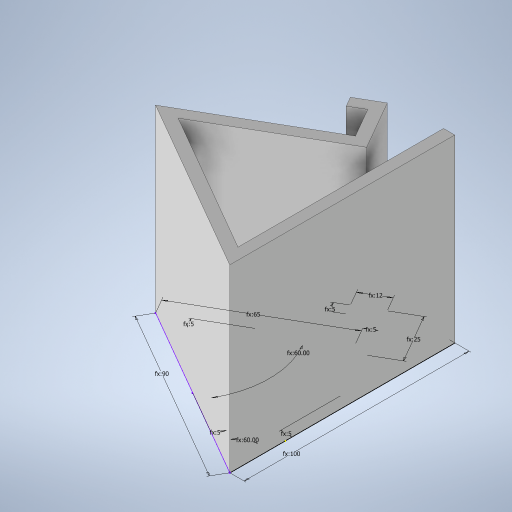
# Autodesk Inventor part: phonestand2DSketch_afterExtrusion
Saved by Autodesk Inventor 2024.2 (Build 282272000, 272)
## iProperties
Created: 2025-02-05
Part Number: phonestand2DSketch_afterExtrusion
Material: Generic
Document SubType Name: Modeling
Designer: veillettem
Density: 1 g/cm^3
Appearance: Default
Author: veillettem
Autodesk Inventor part; units mm, degrees
ref_plane "YZ Plane" through (0, 0, 0) normal (1, 0, 0) x (0, 1, 0)
ref_plane "XZ Plane" through (0, 0, 0) normal (0, 1, 0) x (-1, 0, 0)
ref_plane "XY Plane" through (0, 0, 0) normal (0, 0, 1) x (1, 0, 0)
sketch "PhoneStandProfile" plane through (0, 0, 0) normal (0, 1, 0) x (-1, 0, 0)
  line L0 (5, -75.5038) -> (0, -75.5038)
  line L1 (0, -75.5038) -> (0, 24.4962)
  line L2 (0, 24.4962) -> (77.9423, -20.5038)
  line L3 (77.9423, -20.5038) -> (21.6506, -53.0038)
  line L4 (29.1506, -65.9942) -> (35.2128, -62.4942)
  line L5 (37.7128, -66.8243) -> (27.3205, -72.8243)
  line L6 (27.3205, -72.8243) -> (14.8205, -51.1737)
  line L7 (14.8205, -51.1737) -> (67.9423, -20.5038)
  line L8 (67.9423, -20.5038) -> (5, 15.8359)
  line L9 (5, 15.8359) -> (5, -75.5038)
  line L10 (21.6506, -53.0038) -> (29.1506, -65.9942)
  line L11 (35.2128, -62.4942) -> (37.7128, -66.8243)
  point P0 (0, 0)
  point P1 (0, 24.4962)
  point P2 (77.9423, -20.5038)
  point P3 (5, -29.8339)
  point P4 (38.9711, 1.9962)
  point P5 (49.7965, -36.7538)
  point P6 (21.0705, -61.999)
  point P7 (2.5, -75.5038)
  point P8 (67.9423, -20.5038)
  point P9 (77.9423, -20.5038)
  point P10 (5, 15.8359)
  point P11 (0, 24.4962)
  point P12 (0, 19.6715)
  point P13 (5, 15.8359)
  point P14 (0, 18.7227)
  point P15 (67.9423, -20.5038)
  dimension "angleBackAndSupport" = 60
  dimension "angleBaseAndBack" = 60
  dimension "baseThickness" = 5
  dimension "backThickness" = 5
  dimension "supportThickness" = 5
  dimension "lipThickness" = 5
  dimension "ledgeThickness" = 5
  dimension "ledgeLength" = 25
  dimension "baseL" = 100
  dimension "backL" = 90
  dimension "supportL" = 65
  dimension "lipH" = 12
  constraints: 24 end point, 5 midpoint, 5 point on line, 4 parallel, 4 vertical, 3 perpendicular, 22 other
  measures "angleBackAndSupport" angle of L7 L8
  measures "angleBaseAndBack" angle of L9 L8
  measures "baseThickness" distance from line of L1 point (5, -29.834)
  measures "backThickness" distance from line of L8 point (38.971, 1.996)
  measures "supportThickness" distance from line of point (49.796, -36.754) L7
  measures "lipThickness" distance between parallel lines of L5 L4
  measures "ledgeThickness" distance between parallel lines of L6 L10
  measures "ledgeLength" distance between parallel lines of L5 L7
  measures "baseL" vertical distance of point (0, 24.496) point (2.5, -75.504)
  measures "backL" distance of point (0, 24.496) point (77.942, -20.504)
  measures "supportL" distance of point (77.942, -20.504) L3.end
  measures "lipH" distance of L5.start L5.end
extrude "MainBody" add sketch "PhoneStandProfile" along normal blind 80
sketch "Rectangle" plane through (-37.7128, 0, -66.8243) normal (-0.5, 0, -0.866) x (-0.866, 0, 0.5)
  line L0 (-12, 0) -> (-12, 80) projected
  line L1 (0.2233, 48) -> (-12, 48)
  line L2 (-12, 48) -> (-12, 32)
  line L3 (-12, 32) -> (0.2233, 32)
  line L4 (0.2233, 32) -> (0.2233, 48)
  line L5 (-12, 0) -> (0, 0) projected
  line L6 (-12, 80) -> (0, 80) projected
  point P0 (0.7519, 0)
  point P1 (-6, 80)
  point P2 (-5.8884, 48)
  point P3 (-12, 48)
  dimension "distanceFromRightEdge" = 32
  dimension "distanceFromLeftEdge" = 32
  constraints: 8 end point, 2 midpoint, 2 parallel, 1 horizontal, 1 perpendicular, 1 point on line
  measures "distanceFromRightEdge" distance between parallel lines of L5 L3
  measures "distanceFromLeftEdge" vertical distance of point (-6, 80) point (-5.888, 48)
extrude "CentralNotch" cut sketch "Rectangle" against normal up to surface (20 mm away)
equation "\"angleBackAndSupport\" = internalAngle"
equation "\"angleBaseAndBack\" = internalAngle"
equation "\"baseThickness\" = wallThickness"
equation "\"backThickness\" = wallThickness"
equation "\"supportThickness\" = wallThickness"
equation "\"lipThickness\" = wallThickness"
equation "\"ledgeThickness\" = wallThickness"
equation "\"ledgeLength\" = phoneRestDepth + 2 * wallThickness"
equation "\"baseL\" = baseLength"
equation "\"backL\" = backLength"
equation "\"supportL\" = supportLength"
equation "\"lipH\" = lipHeight"
equation "\"baseW\" = baseWidth"
equation "\"distanceFromRightEdge\" = -0.5 * USBnotchWidth + 0.5 * baseWidth"
equation "\"distanceFromLeftEdge\" = distanceFromRightEdge"
equation "\"d19\" = baseWidth"
equation "\"wallThickness\" = 5"
equation "\"baseLength\" = 100"
equation "\"baseWidth\" = 80"
equation "\"filletRadius\" = 8"
equation "\"internalAngle\" = 60deg"
equation "\"phoneRestDepth\" = 15"
equation "\"USBnotchWidth\" = 16"
equation "\"lipHeight\" = 12"
equation "\"backLength\" = 90"
equation "\"supportLength\" = 65"
body "Solid1"
